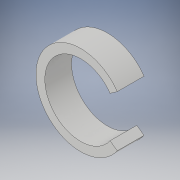
# Autodesk Inventor part: coupler
Saved by Autodesk Inventor 2017 (Build 210142000, 142)
## iProperties
Created: 2018-11-30
Part Number: coupler
Material: Generic
Document SubType Name: Modeling
Designer: ddeboer
Density: 1 g/cm^3
Appearance: Default
Author: ddeboer
Autodesk Inventor part; units mm, degrees
ref_plane "YZ Plane" through (0, 0, 0) normal (1, 0, 0) x (0, 1, 0)
ref_plane "XZ Plane" through (0, 0, 0) normal (0, 1, 0) x (-1, 0, 0)
ref_plane "XY Plane" through (0, 0, 0) normal (0, 0, 1) x (1, 0, 0)
sketch "Sketch1" plane through (0, 0, 0) normal (0, 0, 1) x (1, 0, 0)
  circle A0 centre (0, 0) radius 16.713
  circle A1 centre (0, 0) radius 13.4
  dimension "d0" = 33.426
  dimension "d1" = 26.8
  constraints: 2 centre point, 2 coincident
  measures "d0" diameter of A0
  measures "d1" diameter of A1
extrude "Extrusion1" add sketch "Sketch1" along normal blind 10
sketch "Sketch5" plane through (0, 0, 10) normal (0, 0, 1) x (1, 0, 0)
  line L0 (10.9766, 7.6859) -> (13.6905, 9.5862)
  circle A0 centre (0, 0) radius 16.713 projected
  line L1 (0, 0) -> (16.713, 0) construction
  line L2 (10.9766, -7.6859) -> (13.6905, -9.5862)
  line L3 (0, 0) -> (16.713, 0) construction
  arc A1 (10.9766, -7.6859) -> (10.9766, 7.6859) centre (0, 0) ccw
  dimension "d27" = 35
  dimension "d28" = 35
  constraints: 8 end point, 4 point on circle, 2 horizontal, 1 centre point, 1 coincident
  measures "d27" angle of L1 L0
  measures "d28" angle of L2 L3
extrude "Extrusion5" cut sketch "Sketch5" against normal blind 10 contours L0 A0 L2 A1 picked at (13.3377, 7.9639)
body "Solid1"
